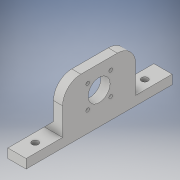
# Autodesk Inventor part: SliderMotorMount
Saved by Autodesk Inventor 2019 (Build 230136000, 136)
## iProperties
Created: 2019-10-06
Part Number: SliderMotorMount
Material: Generic
Document SubType Name: Modeling
Designer: james
Density: 1 g/cm^3
Appearance: Default
Author: james
Autodesk Inventor part; units mm, degrees
ref_plane "YZ Plane" through (0, 0, 0) normal (1, 0, 0) x (0, 1, 0)
ref_plane "XZ Plane" through (0, 0, 0) normal (0, 1, 0) x (-1, 0, 0)
ref_plane "XY Plane" through (0, 0, 0) normal (0, 0, 1) x (1, 0, 0)
sketch "Sketch1" plane through (0, 0, 0) normal (1, 0, 0) x (0, 1, 0)
  line L0 (6.35, 64.4848) -> (0, 64.4848)
  line L1 (0, 64.4848) -> (0, -37.1152)
  line L2 (0, -37.1152) -> (6.35, -37.1152)
  line L3 (38.1, -11.7152) -> (38.1, 39.0848)
  line L4 (38.1, 39.0848) -> (6.35, 39.0848)
  line L5 (38.1, -11.7152) -> (6.35, -11.7152)
  line L6 (6.35, -37.1152) -> (6.35, -11.7152)
  line L7 (6.35, 39.0848) -> (6.35, 64.4848)
  point P0 (0, 0)
  dimension "d1" = 101.6
  dimension "d3" = 25.4
  dimension "d4" = 25.4
  constraints: 16 end point, 3 horizontal, 3 parallel, 1 perpendicular, 1 vertical
  measures "d1" distance of L0.end L1.end
  measures "d3" distance between parallel lines of L5 L2
  measures "d4" distance between parallel lines of L0 L4
extrude "Extrusion1" add sketch "Sketch1" along normal blind 12.7
sketch "Sketch2" plane through (0, 6.35, 64.4848) normal (0, 1, 0) x (1, 0, 0)
  line L0 (0, 0) -> (12.7, 0) projected
  line L1 (12.7, 25.4) -> (12.7, 0) projected
  line L2 (0, 101.6) -> (12.7, 101.6) projected
  line L3 (0, 101.6) -> (0, 76.2) projected
  point P0 (0, 64.4848)
  point P1 (6.35, 12.7)
  point P2 (6.35, 88.9)
  dimension "d7" = 12.7
  dimension "d8" = 6.35
  dimension "d9" = 12.7
  dimension "d10" = 6.35
  measures "d7" distance from line of L0 point (6.35, 12.7)
  measures "d8" distance from line of L1 point (6.35, 12.7)
  measures "d9" distance from line of L2 point (6.35, 88.9)
  measures "d10" distance from line of L3 point (6.35, 88.9)
hole "Hole1" at (6.35, 6.35, 51.7848) at (6.35, 6.35, -24.4152) direction (0, -1, 0) diameter 4.4958 end through all clearance for "Flat Head Machine Screw (82)" size "#8" standard "Ansi Unified Screw Threads"
sketch "Sketch3" plane through (0, 38.1, 39.0848) normal (0, 1, 0) x (1, 0, 0)
  line L0 (-6.071, -5.974) -> (6.35, -5.974)
  line L1 (6.35, -5.974) -> (6.35, 55.8495)
  line L2 (6.35, 55.8495) -> (-6.071, 55.8495)
  line L3 (-6.071, 55.8495) -> (-6.071, -5.974)
  line L4 (0, 50.8) -> (0, 0) projected
  point P0 (0, 39.0848)
  dimension "d18" = 6.35
  constraints: 8 end point, 2 parallel, 1 horizontal, 1 perpendicular
  measures "d18" distance between parallel lines of L4 L1
extrude "Extrusion2" cut sketch "Sketch3" against normal blind 31.75
sketch "Sketch4" plane through (12.7, 0, 0) normal (1, 0, 0) x (0, 0, -1)
  circle A0 centre (-13.6848, 22.225) radius 7.62
  line L0 (11.7152, 38.1) -> (-39.0848, 38.1) projected
  line L1 (11.7152, 6.35) -> (11.7152, 38.1) projected
  point P0 (0, 0)
  dimension "d21" = 15.875
  dimension "d22" = 25.4
  dimension "d25" = 15.24
  constraints: 1 centre point
  measures "d21" distance from line of A0.centre L0
  measures "d22" distance from line of A0.centre L1
  measures "d25" diameter of A0
extrude "Extrusion3" cut sketch "Sketch4" against normal blind 25.4
sketch "Sketch5" plane through (12.7, 0, 0) normal (1, 0, 0) x (0, 0, -1)
  circle A0 centre (-13.6848, 22.225) radius 7.62 projected
  point P0 (0, 0)
  point P1 (-21.6858, 30.226)
  point P2 (-5.6838, 30.226)
  point P3 (-5.6838, 14.224)
  point P4 (-21.6858, 14.224)
  dimension "d26" = 8.001
  dimension "d27" = 8.001
  dimension "d28" = 0
  dimension "d29" = 0
  dimension "d30" = 8.001
  dimension "d31" = 8.001
  dimension "d32" = 0
  dimension "d33" = 0
  measures "d26" horizontal distance of point (-21.686, 30.226) A0.centre
  measures "d27" horizontal distance of A0.centre point (-21.686, 30.226)
  measures "d28" horizontal distance of point (-21.686, 30.226) point (-21.686, 14.224)
  measures "d29" vertical distance of point (-21.686, 30.226) point (-5.684, 30.226)
  measures "d30" horizontal distance of A0.centre point (-5.684, 30.226)
  measures "d31" horizontal distance of A0.centre point (-21.686, 14.224)
  measures "d32" vertical distance of point (-21.686, 14.224) point (-5.684, 14.224)
  measures "d33" horizontal distance of point (-5.684, 14.224) point (-5.684, 30.226)
hole "Hole2" at (12.7, 30.226, 21.6858) at (12.7, 30.226, 5.6838) at (12.7, 14.224, 5.6838) at (12.7, 14.224, 21.6858) direction (-1, 0, 0) diameter 2.4384 end through all clearance for "Flat Head Machine Screw (82)" size "#2" standard "Ansi Unified Screw Threads"
fillet "Fillet1" radius 12.7 2 edges at (9.525, 38.1, 39.0848) (9.525, 38.1, -11.7152)
sketch "Sketch6" plane through (6.35, 6.35, 39.0848) normal (0, 0, 1) x (1, 0, 0)
  line L0 (0, 0) -> (0, 19.05) projected
  line L1 (0, 0) -> (0, 6.35)
  line L2 (0, 6.35) -> (-6.35, 0)
  line L3 (-6.35, 0) -> (0, 0)
  point P0 (-6.35, -6.35)
  dimension "d42" = 45
  constraints: 6 end point, 1 perpendicular, 1 point on line
  measures "d42" angle of L3 L2
extrude "Extrusion4" add sketch "Sketch6" against normal blind 12.7
sketch "Sketch7" plane through (12.7, 6.35, -11.7152) normal (0, 0, -1) x (-1, 0, 0)
  line L0 (6.35, 0) -> (6.35, 19.05) projected
  line L1 (12.7, 0) -> (6.35, 6.35) projected
  line L2 (6.35, 0) -> (12.7, 0)
  line L3 (12.7, 0) -> (6.35, 6.35)
  line L4 (6.35, 6.35) -> (6.35, 0)
  line L5 (4.1021, 0) -> (8.5979, 0) projected
  point P0 (12.7, -6.35)
  constraints: 6 end point, 1 collinear, 1 horizontal, 1 perpendicular
extrude "Extrusion5" add sketch "Sketch7" against normal blind 12.7
body "Solid1"
